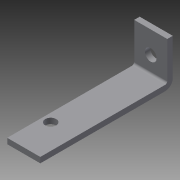
# Autodesk Inventor part: pawl mount
Saved by Autodesk Inventor 2013 (Build 170138000, 138)
## iProperties
Created: 2013-02-05
Part Number: pawl mount
Material: Generic
Document SubType Name: Sheet Metal
Designer: Arpan
Density: 1 g/cm^3
Sheet Metal Rule: Default
Flat Pattern Width: 2.2225 cm
Flat Pattern Length: 13.4488 cm
Flat Pattern Area: 29.8899 cm^2
Sheet Metal Width: 0.875 in
Sheet Metal Length: 5.295 in
Sheet Metal Area: 4.633 in^2
Author: Arpan
Autodesk Inventor part; units mm, degrees
ref_plane "YZ Plane" through (0, 0, 0) normal (1, 0, 0) x (0, 1, 0)
ref_plane "XZ Plane" through (0, 0, 0) normal (0, 1, 0) x (-1, 0, 0)
ref_plane "XY Plane" through (0, 0, 0) normal (0, 0, 1) x (1, 0, 0)
sketch "Sketch1" plane through (0, 0, 0) normal (0, 0, 1) x (1, 0, 0)
  circle A0 centre (9.525, -12.7) radius 3.3782
  line L0 (19.05, 0) -> (0, 0)
  line L1 (0, 0) -> (0, -25.4)
  line L2 (19.05, -25.4) -> (0, -25.4)
  line L3 (19.05, 0) -> (19.05, -25.4)
extrude "Plate1" add sketch "Sketch1" along normal blind 3.175
sketch "Sketch2" plane through (19.05, -22.225, 0) normal (0, -1, 0) x (1, 0, 0)
  line L0 (-19.05, 0) -> (0, 0)
  line L1 (0, 0) -> (0, 25.4)
  line L2 (0, 25.4) -> (-19.05, 25.4)
  line L3 (-19.05, 25.4) -> (-19.05, 0)
  constraints: 6 end point, 1 horizontal, 1 perpendicular, 1 vertical
edge flange "Flange1" height 25.4 angle 90 thickness 3.175 bend radius 1.27 thickness toward (0, -1, 0) relief tear relief width 3.175 relief depth 1.5875 edges at (9.525, -25.4, 3.175) wall of the first edge with corners at (0, -22.225, 0) (19.05, -22.225, 0) (19.05, -22.225, 25.4) (0, -22.225, 25.4)
bend "Bend1"
corner "Corner1"
sketch "Sketch3" plane through (0, -25.4, 25.4) normal (0, 0, 1) x (1, 0, 0)
  line L0 (0, 0) -> (19.05, 0) projected
  line L1 (19.05, 3.175) -> (19.05, 0) projected
  line L2 (0, 3.175) -> (19.05, 3.175) projected
  line L3 (0, 3.175) -> (0, 0) projected
  point P0 (0, 25.4)
extrude "Extrusion1" add sketch "Sketch3" along normal blind 50.8
sketch "Sketch6" plane through (19.05, -25.4, 4.445) normal (0, -1, 0) x (1, 0, 0)
  line L0 (-19.05, 0) -> (-44.45, 0) projected
  circle A0 centre (19.05, 9.8425) radius 38.1 projected
  line L1 (19.05, 51.481) -> (-14.2875, 51.481)
  line L2 (-14.2875, 51.481) -> (19.05, 9.8425)
  circle A1 centre (-14.2875, 51.481) radius 3.175
  point P0 (-19.05, -4.445)
  dimension "d19" = 33.3375
  dimension "d20" = 53.34
  dimension "d21" = 6.35
  constraints: 4 end point, 1 centre point, 1 coincident, 1 parallel, 1 vertical alignment
  measures "d19" distance of L1.start L1.end
  measures "d20" distance of L1.end L2.end
  measures "d21" diameter of A1
extrude "Cut1" cut sketch "Sketch6" against normal blind 3.175 contours A1 L2 L1 | L1 L2 A1
sketch "Sketch7" plane through (0, -25.4, 4.445) normal (-1, 0, 0) x (0, 0, 1)
  line L0 (0, 3.175) -> (0, 0) projected
  arc A0 (-1.27, 4.445) -> (0, 3.175) centre (0, 4.445) ccw projected
  line L1 (-4.445, 4.445) -> (-1.27, 4.445) projected
  arc A1 (-4.445, 4.445) -> (0, 0) centre (0, 4.445) ccw projected
  point P0 (-4.445, 25.4)
sketch "Sketch8" plane through (0, 0, 0) normal (-1, 0, 0) x (0, 0, 1)
  line L0 (0, -20.955) -> (3.175, -20.955) projected
  line L1 (3.175, -20.955) -> (3.175, 0) projected
  line L2 (0, 0) -> (3.175, 0) projected
  line L3 (0, 0) -> (0, -20.955) projected
sketch "Sketch9" plane through (0, -25.4, 4.445) normal (-1, 0, 0) x (0, 0, 1)
  line L0 (0, 3.175) -> (0, 0) projected
  line L1 (0, 0) -> (71.755, 0) projected
  line L2 (71.755, 3.175) -> (71.755, 0) projected
  line L3 (71.755, 3.175) -> (0, 3.175) projected
  point P0 (-4.445, 25.4)
extrude "Extrusion4" add sketch "Sketch8" along normal blind 3.175
extrude "Extrusion5" add sketch "Sketch7" along normal blind 3.175
extrude "Extrusion6" add sketch "Sketch9" along normal blind 3.175
sketch "Sketch10" plane through (0, -25.4, 76.2) normal (0, 0, 1) x (1, 0, 0)
  line L0 (19.05, 0) -> (-3.175, 0) projected
  line L1 (19.05, 0) -> (19.05, 3.175) projected
  line L2 (19.05, 3.175) -> (-3.175, 3.175) projected
  line L3 (-3.175, 0) -> (-3.175, 3.175) projected
  point P0 (0, 25.4)
extrude "Extrusion7" cut sketch "Sketch10" against normal blind 12.7
sketch "Sketch11" plane through (-3.175, -26.67, 64.77) normal (0, 0, 1) x (1, 0, 0)
  line L0 (22.225, 0) -> (0, 0)
  line L1 (0, 0) -> (0, -20.955)
  line L2 (0, -20.955) -> (22.225, -20.955)
  line L3 (22.225, -20.955) -> (22.225, 0)
  constraints: 6 end point, 1 horizontal, 1 perpendicular, 1 vertical
edge flange "Flange2" height 25.4 angle 90 thickness 3.175 bend radius 1.27 thickness toward (0, 0, 1) relief tear relief width 3.175 relief depth 1.5875 edges at (7.9375, -25.4, 63.5) wall of the first edge with corners at (19.05, -26.67, 64.77) (-3.175, -26.67, 64.77) (-3.175, -47.625, 64.77) (19.05, -47.625, 64.77)
bend "Bend2"
corner "Corner2"
sketch "Sketch12" plane through (-3.175, -48.895, 63.5) normal (0, -1, 0) x (1, 0, 0)
  line L0 (22.225, 0) -> (0, 0)
  line L1 (0, 0) -> (0, -20.955)
  line L2 (0, -20.955) -> (22.225, -20.955)
  line L3 (22.225, -20.955) -> (22.225, 0)
  constraints: 6 end point, 1 horizontal, 1 perpendicular, 1 vertical
edge flange "Flange3" height 25.4 angle 90 thickness 3.175 bend radius 1.27 thickness toward (0, -1, 0) relief tear relief width 3.175 relief depth 1.5875 edges at (7.9375, -47.625, 64.77) wall of the first edge with corners at (19.05, -48.895, 63.5) (-3.175, -48.895, 63.5) (-3.175, -48.895, 42.545) (19.05, -48.895, 42.545)
bend "Bend3"
corner "Corner3"
sketch "Sketch13" plane through (-3.175, -52.07, 42.545) normal (0, -1, 0) x (1, 0, 0)
  circle A0 centre (7.9375, 13.381) radius 3.175 projected
  point P0 (3.175, -42.545)
extrude "Cut2" cut sketch "Sketch13" against normal blind 3.175
equation "\"d22\" = Thickness"
equation "\"d52\" = Thickness"
equation "\"d1\" = BendReliefWidth"
equation "\"d2\" = BendReliefDepth"
equation "\"d3\" = MinimumRemnant"
equation "\"d4\" = BendRadius"
equation "\"d8\" = CornerReliefSize"
equation "\"d9\" = GapSize"
equation "\"d10\" = JacobiRadiusSize"
equation "\"d32\" = BendReliefWidth"
equation "\"d33\" = BendReliefDepth"
equation "\"d34\" = MinimumRemnant"
equation "\"d35\" = BendRadius"
equation "\"d39\" = CornerReliefSize"
equation "\"d40\" = GapSize"
equation "\"d41\" = JacobiRadiusSize"
equation "\"d42\" = BendReliefWidth"
equation "\"d43\" = BendReliefDepth"
equation "\"d44\" = MinimumRemnant"
equation "\"d45\" = BendRadius"
equation "\"d49\" = CornerReliefSize"
equation "\"d50\" = GapSize"
equation "\"d51\" = JacobiRadiusSize"
equation "\"BendRadius\" = Thickness"
equation "\"BendReliefWidth\" = Thickness"
equation "\"BendReliefDepth\" = 0.5 * Thickness"
equation "\"CornerReliefSize\" = 4 * Thickness"
equation "\"MinimumRemnant\" = 2 * Thickness"
equation "\"TransitionRadius\" = BendRadius"
equation "\"JacobiRadiusSize\" = Thickness"
equation "\"GapSize\" = Thickness"
equation "\"d0\" = BendRadius"
equation "\"Thickness\" = 3.175"
body "Solid1"
